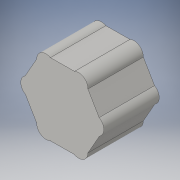
# Autodesk Inventor part: JB_CAD_FinalPt1
Saved by Autodesk Inventor 2016 (Build 200138000, 138)
## iProperties
Created: 2018-06-18
Part Number: JB_CAD_FinalPt1
Material: Generic
Document SubType Name: Modeling
Designer: Student
Density: 1 g/cm^3
Appearance: Default
Author: Student
Autodesk Inventor part; units mm, degrees
ref_plane "YZ Plane" through (0, 0, 0) normal (1, 0, 0) x (0, 1, 0)
ref_plane "XZ Plane" through (0, 0, 0) normal (0, 1, 0) x (-1, 0, 0)
ref_plane "XY Plane" through (0, 0, 0) normal (0, 0, 1) x (1, 0, 0)
sketch "Sketch1" plane through (0, 0, 0) normal (0, 0, 1) x (1, 0, 0)
  line L0 (-11.4295, -0.0912) -> (-11.4381, -0.0912)
  line L1 (-5.798, 9.8601) -> (-5.7937, 9.8528)
  line L2 (5.6401, 9.9513) -> (5.6341, 9.9392)
  line L3 (11.4381, 0.0912) -> (11.4295, 0.0912)
  line L4 (5.798, -9.8601) -> (5.7937, -9.8528)
  line L5 (-5.6401, -9.9513) -> (-5.6341, -9.9392)
  arc A0 (-3.2667, 9.8803) -> (-7.0462, 7.6578) centre (-4.5062, 7.6633) ccw
  arc A1 (7.0443, 7.5633) -> (3.3664, 9.9332) centre (4.5062, 7.6633) ccw
  arc A2 (10.2075, -2.0801) -> (10.1371, 2.3037) centre (8.8895, 0.0912) ccw
  arc A3 (3.2667, -9.8803) -> (7.0462, -7.6578) centre (4.5062, -7.6633) ccw
  arc A4 (-7.0443, -7.5633) -> (-3.3664, -9.9332) centre (-4.5062, -7.6633) ccw
  arc A5 (-10.2075, 2.0801) -> (-10.1371, -2.3037) centre (-8.8895, -0.0912) ccw
  line L6 (-11.4295, -0.1058) -> (-11.4381, -0.0912)
  line L7 (-11.4381, -0.0912) -> (-11.4295, -0.076)
  line L8 (-10.2075, 2.0801) -> (-7.0462, 7.6578)
  line L9 (-5.8064, 9.8453) -> (-5.798, 9.8601)
  line L10 (-5.798, 9.8601) -> (-5.781, 9.8602)
  line L11 (5.6401, 9.9513) -> (5.6527, 9.9298)
  line L12 (-3.2667, 9.8803) -> (3.3664, 9.9332)
  line L13 (5.6098, 9.951) -> (5.6401, 9.9513)
  line L14 (7.0443, 7.5633) -> (10.1371, 2.3037)
  line L15 (11.4295, 0.1058) -> (11.4381, 0.0912)
  line L16 (11.4381, 0.0912) -> (11.4295, 0.076)
  line L17 (10.2075, -2.0801) -> (7.0462, -7.6578)
  line L18 (5.8064, -9.8453) -> (5.798, -9.8601)
  line L19 (5.798, -9.8601) -> (5.781, -9.8602)
  line L20 (-5.6401, -9.9513) -> (-5.6527, -9.9298)
  line L21 (-7.0443, -7.5633) -> (-10.1371, -2.3037)
  line L22 (3.2667, -9.8803) -> (-3.3664, -9.9332)
  line L23 (-5.6098, -9.951) -> (-5.6401, -9.9513)
  point P0 (0, 0)
  constraints: 48 end point, 30 point on circle, 6 centre point, 2 horizontal, 1 parallel, 7 other
extrude "Extrusion1" add sketch "Sketch1" along normal blind 15.24 contours A5 L8 A0 L12 A1 L14 A2 L17 A3 L22 A4 L21
body "Solid1"
